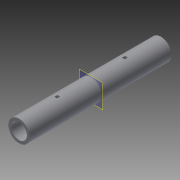
# Autodesk Inventor part: custom pvc spool
Saved by Autodesk Inventor 2013 (Build 170138000, 138)
## iProperties
Created: 2014-01-06
Part Number: custom pvc spool
Material: Generic
Document SubType Name: Modeling
Designer: kahohbein
Density: 1 g/cm^3
Author: kahohbein
Autodesk Inventor part; units mm, degrees
ref_plane "YZ Plane" through (0, 0, 0) normal (1, 0, 0) x (0, 1, 0)
ref_plane "XZ Plane" through (0, 0, 0) normal (0, 1, 0) x (-1, 0, 0)
ref_plane "XY Plane" through (0, 0, 0) normal (0, 0, 1) x (1, 0, 0)
sketch "Sketch1" plane through (0, 0, 0) normal (0, 0, 1) x (1, 0, 0)
  circle A0 centre (0, 0) radius 7.8994
  circle A1 centre (0, 0) radius 10.668
  dimension "d0" = 15.7988
  dimension "d1" = 21.336
  constraints: 2 centre point, 2 coincident
  measures "d0" diameter of A0
  measures "d1" diameter of A1
extrude "Extrusion1" add sketch "Sketch1" along normal blind 141.7574
ref_plane "Work Plane1" through (0, 0, 141.7574) normal (0, 0, 1) x (1, 0, 0)
ref_plane "Work Plane2" through (0, 0, 103.6574) normal (0, 0, 1) x (1, 0, 0)
sketch "Sketch2" plane through (0, 0, 103.6574) normal (0, 0, 1) x (1, 0, 0)
  line L0 (-1.32, 11.5038) -> (1.3938, 11.5038)
  line L1 (1.3938, 11.5038) -> (1.3938, -14.9502)
  line L2 (1.3938, -14.9502) -> (-1.32, -14.9502)
  line L3 (-1.32, -14.9502) -> (-1.32, 11.5038)
  point P0 (0, 0)
  constraints: 8 end point, 2 parallel, 1 horizontal, 1 perpendicular
extrude "Extrusion2" cut sketch "Sketch2" along normal mid plane 3.175
ref_plane "Work Plane3" through (0, 0, 0) normal (0, 0, -1) x (-1, 0, 0)
ref_plane "Work Plane4" through (0, 0, 69.85) normal (0, 0, -1) x (-1, 0, 0)
mirror "Mirror1" about plane through (0, 0, 69.85) normal (0, 0, -1) of "Extrusion2"
body "Solid1"
